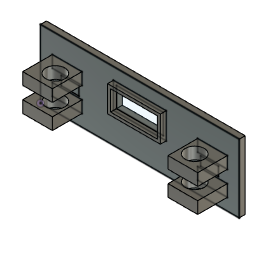
emr2v1 (Autodesk Fusion 360 design; units mm, degrees)
Autodesk Fusion 360 part; units mm, degrees
sketch "Sketch1" plane through (0, 0, 0) normal (0, 1, 0) x (1, 0, 0)
  line L0 (0, 0) -> (33.5, 0)
  line L1 (33.5, 0) -> (33.5, -11.5)
  line L2 (33.5, -11.5) -> (0, -11.5)
  line L3 (0, -11.5) -> (0, 0)
  line L4 (12.8, -9) -> (20.7, -9)
  line L5 (20.7, -9) -> (20.7, -5.6)
  line L6 (20.7, -5.6) -> (12.8, -5.6)
  line L7 (12.8, -5.6) -> (12.8, -9)
  line L8 (12.3, -9.5) -> (21.2, -9.5)
  line L9 (21.2, -9.5) -> (21.2, -5.1)
  line L10 (21.2, -5.1) -> (12.3, -5.1)
  line L11 (12.3, -5.1) -> (12.3, -9.5)
  line L12 (3.5, -5.8) -> (6.5, -5.8)
  line L13 (6.5, -5.8) -> (6.5, -4.3)
  line L14 (6.5, -4.3) -> (3.5, -4.3)
  line L15 (3.5, -4.3) -> (3.5, -5.8)
  line L16 (27, -5.8) -> (30, -5.8)
  line L17 (30, -5.8) -> (30, -4.3)
  line L18 (30, -4.3) -> (27, -4.3)
  line L19 (27, -4.3) -> (27, -5.8)
  line L20 (2, -8.1) -> (7, -8.1)
  line L21 (7, -8.1) -> (7, -6.1)
  line L22 (7, -6.1) -> (2, -6.1)
  line L23 (2, -6.1) -> (2, -8.1)
  line L24 (2, -4) -> (7, -4)
  line L25 (7, -4) -> (7, -2)
  line L26 (7, -2) -> (2, -2)
  line L27 (2, -2) -> (2, -4)
  line L28 (26.5, -8.1) -> (31.5, -8.1)
  line L29 (31.5, -8.1) -> (31.5, -6.1)
  line L30 (31.5, -6.1) -> (26.5, -6.1)
  line L31 (26.5, -6.1) -> (26.5, -8.1)
  line L32 (26.5, -4) -> (31.5, -4)
  line L33 (31.5, -4) -> (31.5, -2)
  line L34 (31.5, -2) -> (26.5, -2)
  line L35 (26.5, -2) -> (26.5, -4)
  dimension "d1" = 7.9
  dimension "d2" = 3.4
  dimension "d3" = 8.9
  dimension "d4" = 4.4
  dimension "d5" = 0.5
  dimension "d6" = 0.5
  dimension "d7" = 3
  dimension "d8" = 1.5
  dimension "d9" = 3
  dimension "d10" = 1.5
  dimension "d12" = 0.2
  dimension "d14" = 0.2
  dimension "d15" = 5
  dimension "d16" = 2
  dimension "d17" = 0.3
  dimension "d18" = 1.5
  dimension "d19" = 5
  dimension "d20" = 2
  dimension "d21" = 1.5
  dimension "d22" = 0.3
  dimension "d23" = 5
  dimension "d24" = 2
  dimension "d25" = 5
  dimension "d26" = 2
  dimension "d27" = 0.5
  dimension "d28" = 0.3
  dimension "d29" = 0.3
  dimension "d30" = 0.5
  dimension "d31" = 2
  dimension "d32" = 2
  dimension "d33" = 2
  dimension "d34" = 2
  dimension "d49" = 20.5
  dimension "d50" = 6.3
  constraint horizontal L0
  constraint vertical L1
  constraint horizontal L2
  constraint vertical L3
  constraint coincident L0.start L3.end
  constraint horizontal L4
  constraint vertical L5
  constraint horizontal L6
  constraint vertical L7
  constraint horizontal L8
  constraint vertical L9
  constraint horizontal L10
  constraint vertical L11
  constraint horizontal L12
  constraint vertical L13
  constraint horizontal L14
  constraint vertical L15
  constraint horizontal L16
  constraint vertical L17
  constraint horizontal L18
  constraint vertical L19
  constraint horizontal L20
  constraint vertical L21
  constraint horizontal L22
  constraint vertical L23
  constraint horizontal L24
  constraint vertical L25
  constraint horizontal L26
  constraint vertical L27
  constraint horizontal L28
  constraint vertical L29
  constraint horizontal L30
  constraint vertical L31
  constraint horizontal L32
  constraint vertical L33
  constraint horizontal L34
  constraint vertical L35
  measures "d1" distance of L4.start L4.end
  measures "d2" distance of L4.start L6.end
  measures "d3" distance of L8.start L8.end
  measures "d4" distance of L8.start L10.end
  measures "d5" distance of L4 L8
  measures "d6" distance of L7 L11
  measures "d7" distance of L12.start L12.end
  measures "d8" distance of L12.start L14.end
  measures "d9" distance of L16.start L16.end
  measures "d10" distance of L16.start L18.end
  measures "d12" distance of L6 L16
  measures "d14" distance of L6 L12
  measures "d15" distance of L20.start L20.end
  measures "d16" distance of L20.start L22.end
  measures "d17" distance of L12 L22
  measures "d18" distance of L15 L23
  measures "d19" distance of L24.start L24.end
  measures "d20" distance of L24.start L26.end
  measures "d21" distance of L15 L27
  measures "d22" distance of L14 L24
  measures "d23" distance of L28.start L28.end
  measures "d24" distance of L28.start L30.end
  measures "d25" distance of L32.start L32.end
  measures "d26" distance of L32.start L34.end
  measures "d27" distance of L19 L31
  measures "d28" distance of L16 L30
  measures "d29" distance of L18 L32
  measures "d30" distance of L19 L35
  measures "d31" distance of L3 L27
  measures "d32" distance of L0 L26
  measures "d33" distance of L1 L29
  measures "d34" distance of L2 L8
  measures "d49" distance of L13 L19
  measures "d50" distance of L7 L13
extrude "Extrude1" add sketch "Sketch1" along normal blind 1 contours L0 L1 L2 L3 | L8 L9 L10 L11 | L12 L13 L14 L15 | L16 L17 L18 L19 | L20 L21 L22 L23 | L24 L25 L26 L27 | L28 L29 L30 L31 | L32 L33 L34 L35
extrude "Extrude2" add sketch "Sketch1" against normal blind 1 contours L8 L9 L10 L11
extrude "Extrude3" add sketch "Sketch1" against normal blind 5 contours L20 L21 L22 L23 | L24 L25 L26 L27 | L28 L29 L30 L31 | L32 L33 L34 L35
sketch "Sketch2" plane through (0, 0, 8.1) normal (0, 0, 1) x (-1, 0, 0)
  line L0 (-7, 0) -> (-2, 0)
  line L1 (-2, 0) -> (-2, 5)
  line L2 (-2, 5) -> (-7, 5)
  line L3 (-7, 5) -> (-7, 0)
  circle A0 centre (-5, 2.5) radius 1.6
  line L4 (-33.5, 0) -> (0, 0)
  circle A1 centre (-28.5, 2.5) radius 1.6
  line L5 (-31.5, 0) -> (-31.5, 5)
  line L6 (-26.5, 0) -> (-26.5, 5)
  dimension "d41" = 3.2
  dimension "d43" = 2.5
  dimension "d44" = 3.2
  dimension "d46" = 2.5
  dimension "d51" = 2
  dimension "d52" = 2
  measures "d41" diameter of A0
  measures "d43" distance of A0.centre L4
  measures "d44" diameter of A1
  measures "d46" distance of L4 A1.centre
  measures "d51" distance of L3 A0.centre
  measures "d52" distance of A1.centre L6
extrude "Extrude4" cut sketch "Sketch2" against normal blind 8 contours A0 | A1
equation "d50 = 5.8 mm + 0.5 mm"
